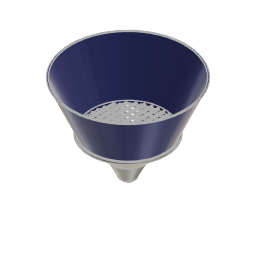
Filter Basket and Funnel Remixed from Klave (Autodesk Fusion 360 design; units mm, degrees)
Autodesk Fusion 360 part; units mm, degrees
note: some values were not read from the file. Set by a fixed rule: which face or edge a step refers to.
sketch "Sketch1" plane through (0, 0, 0) normal (0, 1, 0) x (1, 0, 0)
  line L0 (0, 0) -> (2, 0)
  line L1 (2, 0) -> (2, -1.4)
  line L2 (2, -1.4) -> (0, -1.4)
  line L3 (0, -1.4) -> (0, 0)
  dimension "d13" = 1.4
  dimension "d14" = 2
  constraint horizontal L0
  constraint vertical L1
  constraint horizontal L2
  constraint vertical L3
  constraint coincident L0.start L3.end
  measures "d13" distance of L0.start L2.end
  measures "d14" distance of L0.start L0.end
extrude "Extrude1" add sketch "Sketch1" along normal blind 95 makes body 1
pattern_linear "R-Pattern1" count 15 spacing 6.7857 along (1, 0, 0) of bodies 1 makes body 2 at (7.4524, 31.6667, 0) makes body 3 at (14.2381, 31.6667, 0) makes body 4 at (21.0238, 31.6667, 0) makes body 5 at (27.8095, 31.6667, 0) makes body 6 at (34.5952, 31.6667, 0) makes body 7 at (41.381, 31.6667, 0) makes body 8 at (48.1667, 31.6667, 0) makes body 9 at (54.9524, 31.6667, 0) makes body 10 at (61.7381, 31.6667, 0) makes body 11 at (68.5238, 31.6667, 0) makes body 12 at (75.3095, 31.6667, 0) makes body 13 at (82.0952, 31.6667, 0) makes body 14 at (88.881, 31.6667, 0) makes body 15 at (95.6667, 31.6667, 0)
sketch "Sketch2" plane through (0, 0, 0) normal (-1, 0, 0) x (0, -1, 0)
  line L0 (0, 0) -> (0, 1.4)
  line L1 (0, 1.4) -> (-95, 1.4)
  line L2 (-95, 1.4) -> (-95, 0)
  line L3 (-95, 0) -> (0, 0)
  line L4 (0, 0) -> (-2, 0)
  line L5 (-2, 0) -> (-2, -1.4)
  line L6 (-2, -1.4) -> (0, -1.4)
  line L7 (0, -1.4) -> (0, 0)
  dimension "d19" = 2
  dimension "d20" = 1.4
  constraint horizontal L4
  constraint vertical L5
  constraint horizontal L6
  constraint vertical L7
  constraint coincident L0.start L3.end
  measures "d19" distance of L0.start L4.end
  measures "d20" distance of L0.start L6.end
extrude "Extrude2" add sketch "Sketch2" against normal up to surface (97 mm away) separate body contours L3 L4 L5 L6 L7 makes body 16
pattern_linear "R-Pattern2" count 15 spacing 6.7857 along (0, 1, 0) of bodies 16 makes body 17 at (32.3333, 8.119, -1.4) makes body 18 at (64.6667, 14.9048, -1.4) makes body 19 at (64.6667, 21.6905, -1.4) makes body 20 at (64.6667, 28.4762, -1.4) makes body 21 at (64.6667, 35.2619, -1.4) makes body 22 at (64.6667, 42.0476, -1.4) makes body 23 at (64.6667, 48.8333, -1.4) makes body 24 at (64.6667, 55.619, -1.4) makes body 25 at (64.6667, 62.4048, -1.4) makes body 26 at (64.6667, 69.1905, -1.4) makes body 27 at (64.6667, 75.9762, -1.4) makes body 28 at (64.6667, 82.7619, -1.4) makes body 29 at (64.6667, 89.5476, -1.4) makes body 30 at (64.6667, 96.3333, -1.4)
sketch "Sketch3" plane through (0, 0, 1.4) normal (0, 0, 1) x (-1, 0, 0)
  line L0 (-95, 0) -> (-97, 0)
  line L1 (-97, 0) -> (-97, -95)
  line L2 (-97, -95) -> (-95, -95)
  line L3 (-95, -95) -> (-95, 0)
  line L4 (0, 0) -> (-97, -95) construction
  line L5 (0, -97) -> (-97, 0) construction
  circle A0 centre (-48.5, -48.5) radius 47.5
  point P0 (0, -97)
  dimension "d27" = 95
  constraint coincident L4.start origin
  constraint coincident L1.end L2.start
  constraint coincident L0.end L1.start
  constraint midpoint L5 A0.centre
  constraint coincident P0 L5.start
  measures "d27" diameter of A0
extrude "Extrude3" cut sketch "Sketch3" against normal blind 9 contours L3 A0 | L3 A0 keep common part bodies 1 2 3 4 5 6 7 8 9 10 11 12 13 14 15 16 17 18 19 20 21 22 23 24 25 26 27 28 29 30
combine "Combine1" operation add target body 30 tool bodies 5 22 14 21 13 2 25 1 28 7 12 23 20 15 18 6 17 19 24 3 29 9 11 26 4 8 27 16 10
sketch "Sketch4" plane through (0, 0, 1.4) normal (0, 0, 1) x (-1, 0, 0)
  arc A0 (-2, -58.1954) -> (-2, -38.8046) centre (-48.5, -48.5) ccw
  line L0 (-2, -38.8046) -> (-2, -58.1954)
  arc A1 (-47.5, -1.0105) -> (-49.5, -1.0105) centre (-48.5, -48.5) ccw
  line L1 (-47.5, -95) -> (-47.5, -1.0105)
  line L2 (-49.5, -1.0105) -> (-49.5, -95)
  circle A2 centre (-48.5, -48.5) radius 47.5
  line L3 (-49.5, -95) -> (-47.5, -95)
  dimension "d38" = 95
  constraint coincident A0.centre A1.centre
  measures "d38" diameter of A2
extrude "Extrude4" add sketch "Sketch4" along normal blind 60 draft 24 separate body makes body 31
shell "Shell1" thickness 1.6 removed faces 1 at (28.2728, 47.4957, 61.4) on bodies 31
extrude "Extrude5" cut 1 faces at (52.9893, 42.1949, 3) along direction (0, 0, -1) up to surface (1.6 mm away) on bodies 31 bodies 31
extrude "Extrude6" add 1 faces at (46.4392, 1.8312, 1.4) along direction (0, 0, -1) up to surface (2.8 mm away) on bodies 31 bodies 31
combine "Combine2" operation add target body 31 tool bodies 30
sketch "Sketch5" plane through (0, 0, -1.4) normal (0, 0, -1) x (1, 0, 0)
  arc A0 (81.277, -81.4286) -> (85.4675, -76.6429) centre (48.5, -48.5) ccw
  line L0 (81.277, -81.4286) -> (15.723, -81.4286)
  arc A1 (11.5325, -76.6429) -> (15.723, -81.4286) centre (48.5, -48.5) ccw
  line L1 (11.5325, -76.6429) -> (85.4675, -76.6429)
  arc A2 (4.3832, -63.0714) -> (6.2635, -67.8571) centre (48.5, -48.5) ccw
  line L2 (4.3832, -63.0714) -> (92.6168, -63.0714)
  arc A3 (90.7365, -67.8571) -> (92.6168, -63.0714) centre (48.5, -48.5) ccw
  line L3 (90.7365, -67.8571) -> (6.2635, -67.8571)
  arc A4 (17.8632, -83.4286) -> (24.3879, -88.2143) centre (48.5, -48.5) ccw
  line L4 (17.8632, -83.4286) -> (79.1368, -83.4286)
  arc A5 (72.6121, -88.2143) -> (79.1368, -83.4286) centre (48.5, -48.5) ccw
  line L5 (72.6121, -88.2143) -> (24.3879, -88.2143)
  arc A6 (15.723, -15.5714) -> (11.5325, -20.3571) centre (48.5, -48.5) ccw
  line L6 (15.723, -15.5714) -> (81.277, -15.5714)
  arc A7 (85.4675, -20.3571) -> (81.277, -15.5714) centre (48.5, -48.5) ccw
  line L7 (85.4675, -20.3571) -> (11.5325, -20.3571)
  arc A8 (68.9582, -6.7857) -> (28.0418, -6.7857) centre (48.5, -48.5) ccw
  line L8 (68.9582, -6.7857) -> (28.0418, -6.7857)
  line L9 (24.3879, -8.7857) -> (72.6121, -8.7857)
  arc A9 (79.1368, -13.5714) -> (72.6121, -8.7857) centre (48.5, -48.5) ccw
  line L10 (79.1368, -13.5714) -> (17.8632, -13.5714)
  arc A10 (24.3879, -8.7857) -> (17.8632, -13.5714) centre (48.5, -48.5) ccw
  arc A11 (92.6168, -33.9286) -> (90.7365, -29.1429) centre (48.5, -48.5) ccw
  line L11 (92.6168, -33.9286) -> (4.3832, -33.9286)
  arc A12 (6.2635, -29.1429) -> (4.3832, -33.9286) centre (48.5, -48.5) ccw
  line L12 (6.2635, -29.1429) -> (90.7365, -29.1429)
  line L13 (86.908, -74.6429) -> (10.092, -74.6429)
  arc A13 (7.2387, -69.8571) -> (10.092, -74.6429) centre (48.5, -48.5) ccw
  line L14 (7.2387, -69.8571) -> (89.7613, -69.8571)
  arc A14 (86.908, -74.6429) -> (89.7613, -69.8571) centre (48.5, -48.5) ccw
  arc A15 (2.0498, -49.5) -> (2.4007, -54.2857) centre (48.5, -48.5) ccw
  line L15 (2.0498, -49.5) -> (94.9502, -49.5)
  arc A16 (94.5993, -54.2857) -> (94.9502, -49.5) centre (48.5, -48.5) ccw
  line L16 (94.5993, -54.2857) -> (2.4007, -54.2857)
  line L17 (2.696, -56.2857) -> (94.304, -56.2857)
  arc A17 (93.2278, -61.0714) -> (94.304, -56.2857) centre (48.5, -48.5) ccw
  line L18 (93.2278, -61.0714) -> (3.7722, -61.0714)
  arc A18 (2.696, -56.2857) -> (3.7722, -61.0714) centre (48.5, -48.5) ccw
  arc A19 (2.4007, -42.7143) -> (2.0498, -47.5) centre (48.5, -48.5) ccw
  line L19 (2.4007, -42.7143) -> (94.5993, -42.7143)
  arc A20 (94.9502, -47.5) -> (94.5993, -42.7143) centre (48.5, -48.5) ccw
  line L20 (94.9502, -47.5) -> (2.0498, -47.5)
  arc A21 (3.7722, -35.9286) -> (2.696, -40.7143) centre (48.5, -48.5) ccw
  line L21 (3.7722, -35.9286) -> (93.2278, -35.9286)
  arc A22 (94.304, -40.7143) -> (93.2278, -35.9286) centre (48.5, -48.5) ccw
  line L22 (94.304, -40.7143) -> (2.696, -40.7143)
  line L23 (10.092, -22.3571) -> (86.908, -22.3571)
  arc A23 (89.7613, -27.1429) -> (86.908, -22.3571) centre (48.5, -48.5) ccw
  line L24 (89.7613, -27.1429) -> (7.2387, -27.1429)
  arc A24 (10.092, -22.3571) -> (7.2387, -27.1429) centre (48.5, -48.5) ccw
  circle A25 centre (48.5, -48.5) radius 47.5
  line L25 (28.0418, -90.2143) -> (68.9582, -90.2143)
  arc A26 (28.0418, -90.2143) -> (68.9582, -90.2143) centre (48.5, -48.5) ccw
move_body "Align1" bodies 31 to x (1, 0, 0) y (0, 1, 0) z (0, 0, 1) at (-48.5, -48.5, 1.4)
sketch "Sketch6" plane through (0, 0, 0) normal (0, 1, 0) x (1, 0, 0)
  line L0 (-47.5, 0) -> (-47.5, -2.8)
  line L1 (47.5, -2.8) -> (47.5, 0)
  line L2 (47.7, -0.1739) -> (18.7408, 25)
  line L3 (18.7408, 25) -> (6, 50)
  line L4 (6, 50) -> (9.1597, 46.9396)
  line L5 (9.1597, 46.9396) -> (20.3408, 25)
  line L6 (20.3408, 25) -> (49.3, -0.1739)
  line L7 (49.3, -0.1739) -> (49.3, -2.8)
  line L8 (49.3, -2.8) -> (47.7, -2.8)
  line L9 (-47.5, -2.8) -> (-74.2137, -62.8)
  line L10 (74.2137, -62.8) -> (47.5, -2.8)
  line L11 (0, 0) -> (0, 48.2472) construction
  line L12 (-46.4502, 0) -> (46.4502, 0) construction
  line L13 (47.7, -2.8) -> (47.7, -0.1739)
  dimension "d40" = 41
  dimension "d41" = 1.6
  dimension "d42" = 25
  dimension "d43" = 25
  dimension "d44" = 6
  dimension "d52" = 0.2
  dimension "d53" = 1.6
  constraint parallel L3 L5
  constraint parallel L2 L6
  constraint vertical L7
  constraint horizontal L8
  constraint coincident L11.start origin
  constraint vertical L11
  constraint horizontal L2.end L5.end
  constraint coincident L1.start L8
  constraint perpendicular L8 L13
  constraint coincident L8.end L13.start
  constraint coincident L2.start L13.end
  constraint coincident L1.end L2
  measures "d40" angle of L2 L12
  measures "d41" distance of L2.end L5.end
  measures "d42" distance of L2.end L12
  measures "d43" vertical distance of L2.end L3.end
  measures "d44" horizontal distance of L3.end L11.end
  measures "d52" distance of L1 L13
  measures "d53" distance of L7 L13
revolve "Revolve1" add sketch "Sketch6" angle 360 about axis through (0, 0, 0) along (0, 0, -1) separate body makes body 32
sketch "Sketch7" plane through (0, 0, 0) normal (0, 1, 0) x (1, 0, 0)
  line L0 (9.1597, 46.9396) -> (6, 50)
  line L1 (-6, 50) -> (-9.1597, 46.9396)
  line L2 (20.3408, 25) -> (9.1597, 46.9396)
  line L3 (-9.1597, 46.9396) -> (-20.3408, 25)
  line L4 (6, 50) -> (-15, 41.5)
  line L5 (-15, 41.5) -> (-15, 52)
  line L6 (-15, 52) -> (6, 52)
  line L7 (6, 52) -> (6, 50)
  point P0 (6, 50)
  dimension "d46" = 2
  dimension "d47" = 21
  dimension "d48" = 10.5
  constraint coincident P0 L0.end
  constraint vertical L5
  constraint perpendicular L5 L6
  constraint perpendicular L6 L7
  measures "d46" distance of P0 L6.end
  measures "d47" distance of L5.end L6.end
  measures "d48" distance of L4.end L5.end
extrude "Extrude7" cut sketch "Sketch7" along normal mid plane 62 bodies 32
chamfer "Chamfer1" distance 0.7 angle 45 26 edges at (41.7143, 0, 2.8) (39.7143, 0, 2.8) (34.9286, 0, 2.8) (32.9286, 0, 2.8) (28.1429, 0, 2.8) (26.1429, 0, 2.8) (21.3571, 0, 2.8) (19.3571, 0, 2.8) (14.5714, 0, 2.8) (12.5714, 0, 2.8) (7.7857, 0, 2.8) (5.7857, 0, 2.8) (1, 0, 2.8) (-1, 0, 2.8) (-5.7857, 0, 2.8) (-7.7857, 0, 2.8) (-12.5714, 0, 2.8) (-14.5714, 0, 2.8) (-19.3571, 0, 2.8) (-21.3571, 0, 2.8) (-26.1429, 0, 2.8) (-28.1429, 0, 2.8) (-32.9286, 0, 2.8) (-34.9286, 0, 2.8) (-39.7143, 0, 2.8) (-41.7143, 0, 2.8) on bodies 31
equation "d13 = ( 0.28 * 5 ) * 1 mm"
equation "d19 = d14"
equation "d20 = d13"
equation "d43 = 50 mm - d42"
named bodies: "Sieve", "Filter Basket", "Funnel"
